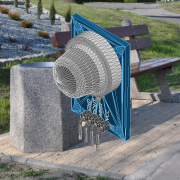
# Autodesk Inventor part: MQ2_1
Saved by Autodesk Inventor 2021 (Build 250183000, 183)
## iProperties
Created: 2025-11-30
Part Number: MQ2_1
Material: Generic
Document SubType Name: Modeling
Designer: huber
Density: 1 g/cm^3
Appearance: Default
Author: huber
Autodesk Inventor part; units mm, degrees
ref_plane "YZ Plane" through (0, 0, 0) normal (1, 0, 0) x (0, 1, 0)
ref_plane "XZ Plane" through (0, 0, 0) normal (0, 1, 0) x (-1, 0, 0)
ref_plane "XY Plane" through (0, 0, 0) normal (0, 0, 1) x (1, 0, 0)
sketch "Sketch1" plane through (-0.395244, -2.23159, 0.595315) normal (0, -0.99923, 0.0392348) x (1, 0, 0)
  line L0 (0.049998, -0.019223) -> (0.049998, 0.050781)
  line L1 (0.049998, 0.050781) -> (-0.019998, 0.050781)
  line L2 (0.03, 0.03) -> (0, 0.03)
  line L3 (0.03, 0) -> (0.03, 0.03)
  line L4 (0, 0) -> (0.03, 0)
  line L5 (0, 0.03) -> (0, 0)
  line L6 (-0.019998, 0.050781) -> (-0.019998, -0.019223)
  line L7 (-0.019998, -0.019223) -> (0.049998, -0.019223)
  line L8 (0.811998, 0.050781) -> (0.742002, 0.050781)
  line L9 (0.811998, -0.019223) -> (0.811998, 0.050781)
  ellipse E0 centre (0.815195, 0.015) end of major axis (0.815195, 0.051066) minor radius 0.025506
  line L10 (0.792, 0.03) -> (0.792, 0)
  line L11 (0.792, 0.03) -> (0.762, 0.03)
  line L12 (0.742002, 0.050781) -> (0.742002, -0.019223)
  line L13 (0.792, 0) -> (0.762, 0)
  line L14 (0.762, 0) -> (0.762, 0.03)
  line L15 (0.742002, -0.019223) -> (0.811998, -0.019223)
  circle A0 centre (0.777, 0.015) radius 0.04895
  line L16 (0.792, 0.03) -> (0.762, 0)
  line L17 (0.762, 0.03) -> (0.792, 0)
  line L18 (0.03, 0.03) -> (0, 0)
  line L19 (0, 0.03) -> (0.03, 0)
  circle A1 centre (0.015, 0.015) radius 0.04895
  point P0 (0.395244, -0.507301)
  constraints: 8 end point, 4 midpoint, 2 perpendicular, 2 point on line, 7 other
sketch "Sketch1 outline for Extrusion1" plane through (-0.395244, -2.23159, 0.595315) normal (0, -0.99923, 0.0392348) x (1, 0, 0)
  circle A0 centre (0.777, 0.015) radius 0.04895
  circle A1 centre (0.015, 0.015) radius 0.04895
extrude "Extrusion1" add sketch "Sketch1 outline for Extrusion1" against normal blind 0.2
body "Solid1"
